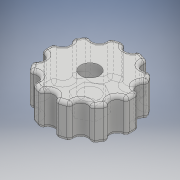
# Autodesk Inventor part: Estrutura - porcaMesa
Saved by Autodesk Inventor 2017 (Build 210142000, 142)
## iProperties
Created: 2020-08-28
Part Number: Estrutura - porcaMesa
Material: Generic
Document SubType Name: Modeling
Designer: ale
Density: 1 g/cm^3
Appearance: Default
Author: ale
Autodesk Inventor part; units mm, degrees
ref_plane "YZ Plane" through (0, 0, 0) normal (1, 0, 0) x (0, 1, 0)
ref_plane "XZ Plane" through (0, 0, 0) normal (0, 1, 0) x (-1, 0, 0)
ref_plane "XY Plane" through (0, 0, 0) normal (0, 0, 1) x (1, 0, 0)
sketch "Sketch1" plane through (0, 0, 0) normal (0, 0, 1) x (1, 0, 0)
  arc A0 (-1.9936, 12.34) -> (1.9936, 12.34) centre (0, 12.5) ccw
  arc A1 (-8.8661, 8.8115) -> (-5.6404, 11.1551) centre (-7.3473, 10.1127) ccw
  arc A2 (-12.3521, 1.9173) -> (-11.12, 5.7093) centre (-11.8882, 3.8627) ccw
  arc A3 (-11.12, -5.7093) -> (-12.3521, -1.9173) centre (-11.8882, -3.8627) ccw
  arc A4 (-5.6404, -11.1551) -> (-8.8661, -8.8115) centre (-7.3473, -10.1127) ccw
  arc A5 (1.9936, -12.34) -> (-1.9936, -12.34) centre (0, -12.5) ccw
  arc A6 (8.8661, -8.8115) -> (5.6404, -11.1551) centre (7.3473, -10.1127) ccw
  arc A7 (12.3521, -1.9173) -> (11.12, -5.7093) centre (11.8882, -3.8627) ccw
  arc A8 (11.12, 5.7093) -> (12.3521, 1.9173) centre (11.8882, 3.8627) ccw
  arc A9 (5.6404, 11.1551) -> (8.8661, 8.8115) centre (7.3473, 10.1127) ccw
  arc A10 (-8.8661, 8.8115) -> (-11.12, 5.7093) centre (0, 0) ccw
  arc A11 (-12.3521, 1.9173) -> (-12.3521, -1.9173) centre (0, 0) ccw
  arc A12 (-11.12, -5.7093) -> (-8.8661, -8.8115) centre (0, 0) ccw
  arc A13 (-5.6404, -11.1551) -> (-1.9936, -12.34) centre (0, 0) ccw
  arc A14 (1.9936, -12.34) -> (5.6404, -11.1551) centre (0, 0) ccw
  arc A15 (8.8661, -8.8115) -> (11.12, -5.7093) centre (0, 0) ccw
  arc A16 (12.3521, -1.9173) -> (12.3521, 1.9173) centre (0, 0) ccw
  arc A17 (11.12, 5.7093) -> (8.8661, 8.8115) centre (0, 0) ccw
  arc A18 (5.6404, 11.1551) -> (1.9936, 12.34) centre (0, 0) ccw
  arc A19 (-1.9936, 12.34) -> (-5.6404, 11.1551) centre (0, 0) ccw
  dimension "d1" = 4
  dimension "d4" = 360
  constraints: 40 point on circle, 20 centre point, 1 coincident, 41 other
  measures "d1" diameter of A0
extrude "Extrusion1" add sketch "Sketch1" along normal blind 10
sketch "Sketch2" plane through (0, 0, 10) normal (0, 0, 1) x (1, 0, 0)
  circle A0 centre (0, 0) radius 2.75
  dimension "d8" = 5.5
  constraints: 1 centre point, 1 coincident
  measures "d8" diameter of A0
hole "Hole1" at (0, 0, 10) direction (0, 0, -1) diameter 5.5 end through all
sketch "Sketch3" plane through (0, 0, 0) normal (0, 0, -1) x (-1, 0, 0)
  line L0 (0, -4.5) -> (-3.8971, -2.25)
  line L1 (-3.8971, -2.25) -> (-3.8971, 2.25)
  line L2 (-3.8971, 2.25) -> (0, 4.5)
  line L3 (0, 4.5) -> (3.8971, 2.25)
  line L4 (3.8971, 2.25) -> (3.8971, -2.25)
  line L5 (3.8971, -2.25) -> (0, -4.5)
  point P0 (0, 0)
  point P1 (0, 0)
  dimension "d16" = 9
  constraints: 12 end point, 1 coincident, 13 other
  measures "d16" distance of L0.start L2.end
extrude "Extrusion2" cut sketch "Sketch3" against normal blind 4
fillet "Fillet1" radius 1 60 edges at (3.8627, 11.8882, 0) (1.9936, 12.34, 5) (3.8627, 11.8882, 10) (5.6404, 11.1551, 5) (6.1717, 8.4947, 0) (6.1717, 8.4947, 10) (8.8661, 8.8115, 5) (10.1127, 7.3473, 0) (10.1127, 7.3473, 10) (11.12, 5.7093, 5) (9.9861, 3.2447, 0) (9.9861, 3.2447, 10) (12.3521, 1.9173, 5) (12.5, 0, 0) (12.5, 0, 10) (12.3521, -1.9173, 5) (9.9861, -3.2447, 0) (9.9861, -3.2447, 10) (11.12, -5.7093, 5) (10.1127, -7.3473, 0) (10.1127, -7.3473, 10) (8.8661, -8.8115, 5) (6.1717, -8.4947, 0) (6.1717, -8.4947, 10) (5.6404, -11.1551, 5) (3.8627, -11.8882, 0) (3.8627, -11.8882, 10) (1.9936, -12.34, 5) (0, -10.5, 0) (0, -10.5, 10) (-1.9936, -12.34, 5) (-3.8627, -11.8882, 0) (-3.8627, -11.8882, 10) (-5.6404, -11.1551, 5) (-6.1717, -8.4947, 0) (-6.1717, -8.4947, 10) (-8.8661, -8.8115, 5) (-10.1127, -7.3473, 0) (-10.1127, -7.3473, 10) (-11.12, -5.7093, 5) (-9.9861, -3.2447, 0) (-9.9861, -3.2447, 10) (-12.3521, -1.9173, 5) (-12.5, 0, 0) (-12.5, 0, 10) (-12.3521, 1.9173, 5) (-9.9861, 3.2447, 0) (-9.9861, 3.2447, 10) (-11.12, 5.7093, 5) (-10.1127, 7.3473, 0) (-10.1127, 7.3473, 10) (-8.8661, 8.8115, 5) (-6.1717, 8.4947, 0) (-6.1717, 8.4947, 10) (-5.6404, 11.1551, 5) (-3.8627, 11.8882, 0) (-3.8627, 11.8882, 10) (-1.9936, 12.34, 5) (0, 10.5, 0) (0, 10.5, 10)
body "Solid1"
